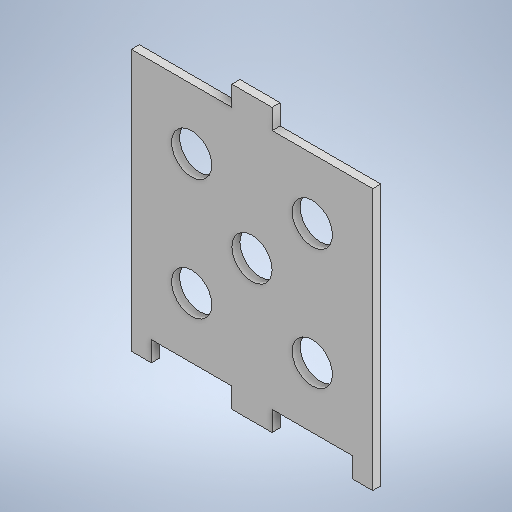
# Autodesk Inventor part: Middle Air Layer
Saved by Autodesk Inventor 2025.1 (Build 291241020, 241B)
## iProperties
Created: 2024-10-29
Part Number: Middle Air Layer
Material: Generic
Document SubType Name: Modeling
Designer: jjk
Density: 1 g/cm^3
Appearance: Default
Author: jjk
Autodesk Inventor part; units mm, degrees
ref_plane "YZ Plane" through (0, 0, 0) normal (1, 0, 0) x (0, 1, 0)
ref_plane "XZ Plane" through (0, 0, 0) normal (0, 1, 0) x (-1, 0, 0)
ref_plane "XY Plane" through (0, 0, 0) normal (0, 0, 1) x (1, 0, 0)
sketch "Sketch1" plane through (0, 0, 0) normal (0, 0, 1) x (1, 0, 0)
  line L0 (0, 0) -> (152.4, 0)
  line L1 (152.4, 0) -> (152.4, 152.4)
  line L2 (0, 152.4) -> (0, 0)
  line L3 (88.9, 152.4) -> (88.9, 165.1)
  line L4 (88.9, 165.1) -> (76.2, 165.1)
  line L5 (76.2, 165.1) -> (63.5, 165.1)
  line L6 (63.5, 165.1) -> (63.5, 152.4)
  line L7 (152.4, 152.4) -> (88.9, 152.4)
  line L8 (63.5, 152.4) -> (0, 152.4)
  circle A0 centre (38.1, 114.3) radius 12.7
  circle A1 centre (114.3, 114.3) radius 12.7
  circle A2 centre (76.2, 76.2) radius 12.7
  circle A3 centre (38.1, 38.1) radius 12.7
  circle A4 centre (114.3, 38.1) radius 12.7
  line L9 (63.5, 152.4) -> (63.5, -12.7)
  line L10 (88.9, 152.4) -> (88.9, -12.7)
  line L11 (63.5, 0) -> (88.9, 0)
  line L12 (88.9, 0) -> (88.9, -12.7)
  line L13 (88.9, -12.7) -> (63.5, -12.7)
  line L14 (63.5, -12.7) -> (63.5, 0)
  dimension "d0" = 152.4
  dimension "d1" = 152.4
  dimension "d5" = 12.7
  dimension "d6" = 12.7
  dimension "d7" = 12.7
  dimension "d8" = 12.7
  dimension "d9" = 63.5
  dimension "d10" = 90
  dimension "d11" = 25.4
  dimension "d12" = 25.4
  dimension "d13" = 25.4
  dimension "d14" = 25.4
  dimension "d15" = 25.4
  dimension "d16" = 38.1
  dimension "d17" = 38.1
  dimension "d18" = 38.1
  dimension "d19" = 38.1
  dimension "d20" = 76.2
  dimension "d21" = 76.2
  dimension "d22" = 38.1
  dimension "d23" = 38.1
  dimension "d24" = 38.1
  dimension "d25" = 38.1
  dimension "d26" = 12.7
  constraints: 30 end point, 5 centre point, 5 parallel, 3 horizontal, 3 perpendicular, 2 point on line, 2 vertical
  measures "d0" distance of L0.end L1.end
  measures "d1" distance of L1.end L2.start
  measures "d5" distance of L3.end L4.end
  measures "d6" distance of L4.end L5.end
  measures "d7" distance of L3.start L3.end
  measures "d8" distance of L5.end L6.end
  measures "d9" distance of L6.end L2.start
  measures "d10" angle of L3 L4
  measures "d11" diameter of A0
  measures "d12" diameter of A1
  measures "d13" diameter of A2
  measures "d14" diameter of A3
  measures "d15" diameter of A4
  measures "d16" distance from line of L2 A0.centre
  measures "d17" distance from line of L8 A0.centre
  measures "d18" distance from line of L7 A1.centre
  measures "d19" distance from line of L1 A1.centre
  measures "d20" distance from line of L1 A2.centre
  measures "d21" distance from line of L8 A2.centre
  measures "d22" distance from line of L2 A3.centre
  measures "d23" distance from line of L1 A4.centre
  measures "d24" distance from line of L0 A4.centre
  measures "d25" distance from line of L0 A3.centre
  measures "d26" distance of L11.end L10.end
extrude "Extrusion1" add sketch "Sketch1" along normal blind 5.08 contours L2 L8 L9 L0 | L9 A2 L10 L0 | L0 L10 L13 L9 | L10 L7 L1 L0 | L9 L6 L5 L4 L3 L10 A2
sketch "Sketch2" plane through (0, 0, 0) normal (0, -1, 0) x (1, 0, 0)
  line L0 (63.5, 5.08) -> (0, 5.08) projected
  line L1 (0, 0) -> (12.7, 0)
  line L2 (12.7, 0) -> (12.7, 5.08)
  line L3 (12.7, 5.08) -> (0, 5.08)
  line L4 (0, 5.08) -> (0, 0)
  line L5 (88.9, 5.08) -> (152.4, 5.08) projected
  line L6 (152.4, 0) -> (139.7, 0)
  line L7 (139.7, 0) -> (139.7, 5.08)
  line L8 (139.7, 5.08) -> (152.4, 5.08)
  line L9 (152.4, 5.08) -> (152.4, 0)
  dimension "d29" = 12.7
  dimension "d31" = 12.7
  constraints: 16 end point, 4 parallel, 2 horizontal, 2 perpendicular, 2 point on line
  measures "d29" distance between parallel lines of L4 L2
  measures "d31" distance between parallel lines of L9 L7
extrude "Extrusion2" add sketch "Sketch2" along normal blind 12.7
body "Solid1"
